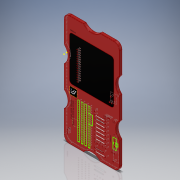
# Autodesk Inventor part: M5 Stack
Saved by Autodesk Inventor 2019 (Build 230136000, 136)
## iProperties
Created: 2020-01-20
Part Number: M5 Stack
Material: PET Plastic
Document SubType Name: Modeling
Designer: Leonardo
Density: 1.541 g/cm^3
Appearance: Red
Mass: 0.203324 g
Surface Area: 4.56566 cm^2
Volume: 0.199142 cm^3
Author: Leonardo
Autodesk Inventor part; units mm, degrees
(part 1 of 2)
ref_plane "YZ Plane" through (0, 0, 0) normal (1, 0, 0) x (0, 1, 0)
ref_plane "XZ Plane" through (0, 0, 0) normal (0, 1, 0) x (-1, 0, 0)
ref_plane "XY Plane" through (0, 0, 0) normal (0, 0, 1) x (1, 0, 0)
sketch "Sketch1" plane through (0, 0, 0) normal (0, 0, 1) x (1, 0, 0)
  line L0 (1, 6.5) -> (9, 6.5)
  line L1 (10, 5.5) -> (10, -12.5)
  line L2 (9, -13.5) -> (1, -13.5)
  line L3 (0, -12.5) -> (0, 5.5)
  arc A0 (10, 5.5) -> (9, 6.5) centre (9, 5.5) ccw
  arc A1 (1, 6.5) -> (0, 5.5) centre (1, 5.5) ccw
  arc A2 (0, -12.5) -> (1, -13.5) centre (1, -12.5) ccw
  arc A3 (9, -13.5) -> (10, -12.5) centre (9, -12.5) ccw
  point P0 (0, 0)
  point P1 (0, 6.5)
  point P2 (10, -13.5)
  point P3 (10, 6.5)
  point P4 (0, -13.5)
  dimension "d0" = 10
  dimension "d1" = 20
  dimension "d5" = 1
  dimension "d6" = 1
  dimension "d7" = 1
  constraints: 8 end point, 8 point on circle, 8 point on line, 8 tangent, 4 centre point, 2 parallel, 1 equal radius, 1 horizontal, 1 perpendicular
  measures "d0" distance of point (0, 6.5) point (10, 6.5)
  measures "d1" distance of point (10, 6.5) point (10, -13.5)
  measures "d5" radius of A0
  measures "d6" radius of A1
  measures "d7" radius of A2
extrude "Extrusion1" add sketch "Sketch1" along normal blind 0.5
sketch "Sketch3" plane through (0, 0, 0.5) normal (0, 0, 1) x (1, 0, 0)
  arc A0 (1, 6.5) -> (0, 5.5) centre (1, 5.5) ccw projected
  line L0 (1, 4) -> (9, 4)
  line L1 (9, 4) -> (9, -4.5)
  line L2 (9, -4.5) -> (1, -4.5)
  line L3 (1, -4.5) -> (1, 4)
  line L4 (9, -13.5) -> (1, -13.5) projected
  line L5 (5, -13.5) -> (5, -6)
  circle A1 centre (7.5, -6.0106) radius 0.0625
  line L6 (7.5, -6.0106) -> (7.5, -6.2106)
  line L7 (0, 5.5) -> (0, -12.5) projected
  line L8 (0, -3.5) -> (10.2754, -3.5)
  circle A2 centre (7.5, -6.2106) radius 0.0625
  line L9 (7.5, -6.2106) -> (7.5, -6.7106)
  circle A3 centre (7.5, -6.7106) radius 0.0625
  line L10 (7.5, -6.7106) -> (7.5, -7.2106)
  circle A4 centre (7.5, -7.2106) radius 0.0625
  circle A5 centre (7.5, -7.8356) radius 0.0625
  circle A6 centre (7.5, -8.4606) radius 0.0625
  circle A7 centre (7.5, -9.0856) radius 0.0625
  circle A8 centre (7.5, -9.7106) radius 0.0625
  circle A9 centre (7.5, -10.3356) radius 0.0625
  circle A10 centre (7.5, -10.9606) radius 0.0625
  line L11 (7.5, -5.9481) -> (5.5, -5.9481)
  line L12 (6.5, -5.9481) -> (6.5, -13.5)
  circle A11 centre (5.5, -6.0106) radius 0.0625
  line L13 (5.5, -6.0106) -> (5.5, -6.2106)
  circle A12 centre (5.5, -6.2106) radius 0.0625
  line L14 (5.5, -6.2106) -> (5.5, -6.7106)
  circle A13 centre (5.5, -6.7106) radius 0.0625
  line L15 (5.5, -6.7106) -> (5.5, -7.2106)
  circle A14 centre (5.5, -7.2106) radius 0.0625
  circle A15 centre (5.5, -7.8356) radius 0.0625
  line L16 (5.5, -7.7106) -> (5.5, -8.4606)
  circle A16 centre (5.5, -8.4606) radius 0.0625
  line L17 (5.5, -8.3356) -> (5.5, -9.0856)
  circle A17 centre (5.5, -9.0856) radius 0.0625
  line L18 (5.5, -8.9606) -> (5.5, -9.7106)
  circle A18 centre (5.5, -9.7106) radius 0.0625
  line L19 (5.5, -9.5856) -> (5.5, -10.3356)
  circle A19 centre (5.5, -10.3356) radius 0.0625
  line L20 (5.5, -10.2106) -> (5.5, -10.9606)
  circle A20 centre (5.5, -10.9606) radius 0.0625
  line L21 (5.5, -5.9481) -> (7.5, -5.9481)
  circle A21 centre (7.5, -12.3356) radius 0.0625
  circle A22 centre (5.5, -12.3356) radius 0.0625
  line L22 (7.5, -11.7731) -> (7.1, -11.7731)
  line L23 (7.5, -11.7731) -> (7.9, -11.7731) construction
  circle A23 centre (7.1, -11.7731) radius 0.0625
  line L24 (5.5, -10.9606) -> (5.5, -12.3782)
  line L25 (7.5, -11.0231) -> (7.7613, -11.0231)
  circle A24 centre (5.5, -11.7731) radius 0.0625
  circle A25 centre (6.5, -10.9606) radius 0.0625
  circle A26 centre (7, -10.9606) radius 0.0625
  circle A27 centre (6, -10.9606) radius 0.0625
  point P0 (0, 0)
  dimension "d10" = 0.125
  dimension "d35" = 0.125
  dimension "d8" = 7.5
  dimension "d11" = 0.2
  dimension "d12" = 0.125
  dimension "d13" = 1
  dimension "d14" = 8.5
  dimension "d15" = 8
  dimension "d16" = 0.5
  dimension "d17" = 0.125
  dimension "d18" = 0.5
  dimension "d19" = 0.125
  dimension "d23" = 0.125
  dimension "d25" = 0.125
  dimension "d27" = 0.125
  dimension "d29" = 0.125
  dimension "d31" = 0.125
  dimension "d38" = 2
  dimension "d64" = 0.5
  dimension "d65" = 0.5
  dimension "d66" = 0.5
  dimension "d67" = 0.5
  dimension "d68" = 0.5
  dimension "d69" = 0.5
  dimension "d70" = 0.125
  dimension "d71" = 1.25
  dimension "d72" = 180
  dimension "d73" = 0.125
  dimension "d75" = 0.4
  dimension "d78" = 0.75
  dimension "d79" = 0.125
  dimension "d80" = 0.125
  dimension "d81" = 0.125
  dimension "d82" = 0.125
  constraints: 48 end point, 24 centre point, 16 symmetric about line, 12 coincident, 6 vertical, 5 horizontal, 3 midpoint, 3 vertical alignment, 2 parallel, 2 perpendicular, 2 point on line, 1 collinear, 16 other
  measures "d8" distance of L5.start L5.end
  measures "d11" distance of L6.start L6.end
  measures "d12" diameter of A2
  measures "d13" distance from line of L7 L0.start
  measures "d14" distance from line of L2 L0.end
  measures "d15" distance of L0.end L0.start
  measures "d16" distance of L9.start L9.end
  measures "d17" diameter of A3
  measures "d18" distance of L10.start L10.end
  measures "d19" diameter of A4
  measures "d23" diameter of A5
  measures "d25" diameter of A6
  measures "d27" diameter of A7
  measures "d29" diameter of A8
  measures "d31" diameter of A9
  measures "d38" distance of L11.start L11.end
  measures "d70" diameter of A21
  measures "d72" angle of L22 L23
  measures "d73" diameter of A23
  measures "d75" distance of L22.end L22.start
  measures "d78" distance from line of L22.start L25
  measures "d79" diameter of A24
  measures "d80" diameter of A25
  measures "d81" diameter of A26
  measures "d82" diameter of A27
sketch "Sketch4" plane through (0, 0, 0.5) normal (0, 0, 1) x (1, 0, 0)
  line L0 (0, 5.5) -> (0, -12.5) projected
  line L1 (0, -3.5) -> (14.3961, -3.5)
  circle A0 centre (7.5, -8.4606) radius 0.0625 projected
  circle A1 centre (7.5, -6.0106) radius 0.0625 projected
  line L2 (7.5, -6.0106) -> (10.4645, -6.0106)
  line L3 (7.5, -6.0106) -> (10.4645, -6.0106) construction
  circle A2 centre (7.725, -6.0106) radius 0.0625
  circle A3 centre (7.95, -6.0106) radius 0.0625
  circle A4 centre (8.095, -6.0106) radius 0.0625
  circle A5 centre (8.24, -6.0106) radius 0.0625
  circle A6 centre (8.865, -6.0106) radius 0.0625
  circle A7 centre (9.09, -6.0106) radius 0.0625
  line L4 (9.09, -6.0106) -> (9.09, -8.5018)
  line L5 (9.09, -6.0106) -> (11.5812, -6.0106) construction
  circle A8 centre (9.09, -8.5018) radius 0.125
  line L6 (9.09, -8.5018) -> (9.09, -10.8899)
  line L7 (9.09, -8.5018) -> (11.4781, -8.5018) construction
  circle A9 centre (9.09, -8.9993) radius 0.0625
  circle A10 centre (9.09, -9.4343) radius 0.0625
  circle A11 centre (9.09, -9.8693) radius 0.0625
  circle A12 centre (9.09, -10.3668) radius 0.125
  line L8 (9.09, -10.8899) -> (9.09, -11.0971)
  line L9 (10, -12.5) -> (10, 5.5) projected
  circle A13 centre (9.0887, -11.003) radius 0.1
  circle A14 centre (8.6887, -11.003) radius 0.1
  line L10 (7.5, -12.3316) -> (9.6048, -12.3316)
  line L11 (7.5, -12.3316) -> (9.6048, -12.3316) construction
  line L12 (8.89, -11.003) -> (9.29, -11.003)
  circle A15 centre (8.8887, -12.3316) radius 0.1
  point P0 (0, 0)
  dimension "d41" = 0.125
  dimension "d42" = 0.1
  dimension "d43" = 0.125
  dimension "d44" = 0.125
  dimension "d45" = 0.125
  dimension "d46" = 0.1
  dimension "d47" = 0.02
  dimension "d48" = 0.02
  dimension "d49" = 0.125
  dimension "d50" = 0.125
  dimension "d51" = 0.1
  dimension "d52" = 0.5
  dimension "d53" = 90
  dimension "d54" = 0.25
  dimension "d55" = 90
  dimension "d56" = 0.125
  dimension "d57" = 0.125
  dimension "d58" = 0.125
  dimension "d59" = 0.25
  dimension "d60" = 0.31
  dimension "d61" = 0.31
  dimension "d62" = 0.31
  dimension "d63" = 0.31
  dimension "d84" = 0.2
  dimension "d86" = 0.2
  dimension "d87" = 0.2
  dimension "d90" = 0.2
  constraints: 22 end point, 14 centre point, 10 point on line, 6 horizontal, 4 equal length, 1 coincident, 1 midpoint, 1 parallel
  measures "d41" diameter of A2
  measures "d43" diameter of A3
  measures "d44" diameter of A4
  measures "d45" diameter of A5
  measures "d49" diameter of A6
  measures "d50" diameter of A7
  measures "d53" angle of L4 L5
  measures "d54" diameter of A8
  measures "d55" angle of L6 L7
  measures "d56" diameter of A9
  measures "d57" diameter of A10
  measures "d58" diameter of A11
  measures "d59" diameter of A12
  measures "d84" diameter of A13
  measures "d86" diameter of A14
  measures "d90" diameter of A15
extrude "Extrusion3" cut sketch "Sketch3" against normal blind 2 contours A1 | A4 | A3 L10 L9 | L9 L10 A3 | A2 L9 L6 | L6 L9 A2 | A25 L12 | L12 A25 | A14 | A13 L15 L14 | L14 L15 A13 | A12 L14 L13 | L13 L14 A12 | A11 | A5 | A6 | A7 | A8 | A9 | A10 | A15 L16 | A22 | A20 L24 L20 | L20 L24 A20 | A19 L20 L19 | L19 L20 A19 | A18 L19 L18 | L18 L19 A18 | A17 L18 L17 | L17 L18 A17 | A16 L17 L16 | L16 L17 A16 | L16 A15 | A21 | A23 | A26 | A27
extrude "Extrusion4" cut sketch "Sketch4" against normal blind 2 contours A13 L12 L8 | L8 L12 A13 | A12 L6 | L6 A12 | A11 L6 | L6 A11 | A10 L6 | L6 A10 | A9 L6 | L6 A9 | A8 L6 L4 | L4 L6 A8 | A7 L2 | L2 L4 A7 | A6 L2 | L2 A6 | A5 L2 | L2 A5 | A4 L2 | L2 A4 | A3 L2 | L2 A3 | A2 L2 | L2 A2 | L2 A7 L4 | L12 A13 | A14 | A15 L10 | L10 A15
sketch "Sketch5" plane through (0, 0, 0.5) normal (0, 0, 1) x (1, 0, 0)
  line L0 (0, -12.5) -> (10, -12.5)
  line L1 (0, -12.5) -> (10, -12.5) construction
  line L2 (5, -12.5) -> (5, -4)
  line L3 (5, -12.5) -> (2.2, -12.5)
  line L4 (2.2, -12.5) -> (2.2, -5.5)
  line L5 (2.2, -5.5) -> (2.2, -6)
  circle A0 centre (2.625, -6) radius 0.0625
  circle A1 centre (3.25, -6) radius 0.0625
  circle A2 centre (3.875, -6) radius 0.0625
  circle A3 centre (4.5, -6) radius 0.0625
  line L6 (2.625, -6) -> (2.625, -12.5)
  line L7 (2.625, -6) -> (9.125, -6) construction
  line L8 (2.625, -6.36) -> (2.9536, -6.36)
  line L9 (2.625, -6.72) -> (2.9536, -6.72)
  line L10 (2.625, -7.08) -> (3, -7.08)
  line L11 (2.625, -8.16) -> (3.0688, -8.16)
  line L12 (2.625, -8.52) -> (2.9536, -8.52)
  line L13 (2.625, -8.88) -> (3.3125, -8.88)
  line L14 (2.625, -9.24) -> (3.1875, -9.24)
  line L15 (2.625, -9.6) -> (3.25, -9.6)
  line L16 (2.625, -9.96) -> (3.3913, -9.96)
  line L17 (2.625, -10.32) -> (3.3125, -10.32)
  line L18 (2.625, -10.68) -> (3.1226, -10.68)
  line L19 (2.625, -11.04) -> (3.1226, -11.04)
  line L20 (2.625, -11.4) -> (3.1875, -11.4)
  line L21 (2.625, -11.76) -> (3.25, -11.76)
  line L22 (2.625, -12.12) -> (3.1875, -12.12)
  line L23 (2.625, -7.44) -> (3.0082, -7.44)
  line L24 (2.625, -7.8) -> (3.1226, -7.8)
  circle A4 centre (2.625, -6.36) radius 0.0625
  circle A5 centre (3.25, -6.36) radius 0.0625
  circle A6 centre (3.875, -6.36) radius 0.0625
  circle A7 centre (4.5, -6.36) radius 0.0625
  circle A8 centre (2.625, -6.72) radius 0.0625
  circle A9 centre (3.25, -6.72) radius 0.0625
  circle A10 centre (3.875, -6.72) radius 0.0625
  circle A11 centre (4.5, -6.72) radius 0.0625
  circle A12 centre (2.625, -7.08) radius 0.0625
  circle A13 centre (3.25, -7.08) radius 0.0625
  circle A14 centre (3.875, -7.08) radius 0.0625
  circle A15 centre (4.5, -7.08) radius 0.0625
  circle A16 centre (2.625, -7.44) radius 0.0625
  circle A17 centre (3.25, -7.44) radius 0.0625
  circle A18 centre (3.875, -7.44) radius 0.0625
  circle A19 centre (4.5, -7.44) radius 0.0625
  circle A20 centre (2.625, -7.8) radius 0.0625
  circle A21 centre (3.25, -7.8) radius 0.0625
  circle A22 centre (3.875, -7.8) radius 0.0625
  circle A23 centre (4.5, -7.8) radius 0.0625
  circle A24 centre (2.625, -8.16) radius 0.0625
  circle A25 centre (3.25, -8.16) radius 0.0625
  circle A26 centre (3.875, -8.16) radius 0.0625
  circle A27 centre (4.5, -8.16) radius 0.0625
  circle A28 centre (2.625, -8.52) radius 0.0625
  circle A29 centre (3.25, -8.52) radius 0.0625
  circle A30 centre (3.875, -8.52) radius 0.0625
  circle A31 centre (4.5, -8.52) radius 0.0625
  circle A32 centre (2.625, -8.88) radius 0.0625
  circle A33 centre (3.25, -8.88) radius 0.0625
  circle A34 centre (3.875, -8.88) radius 0.0625
  circle A35 centre (4.5, -8.88) radius 0.0625
  circle A36 centre (2.625, -9.24) radius 0.0625
  circle A37 centre (3.25, -9.24) radius 0.0625
  circle A38 centre (3.875, -9.24) radius 0.0625
  circle A39 centre (4.5, -9.24) radius 0.0625
  circle A40 centre (2.625, -9.6) radius 0.0625
  circle A41 centre (3.25, -9.6) radius 0.0625
  circle A42 centre (3.875, -9.6) radius 0.0625
  circle A43 centre (4.5, -9.6) radius 0.0625
  circle A44 centre (2.625, -9.96) radius 0.0625
  circle A45 centre (3.25, -9.96) radius 0.0625
  circle A46 centre (3.875, -9.96) radius 0.0625
  circle A47 centre (4.5, -9.96) radius 0.0625
  circle A48 centre (2.625, -10.32) radius 0.0625
  circle A49 centre (3.25, -10.32) radius 0.0625
  circle A50 centre (3.875, -10.32) radius 0.0625
  circle A51 centre (4.5, -10.32) radius 0.0625
  circle A52 centre (2.625, -10.68) radius 0.0625
  circle A53 centre (3.25, -10.68) radius 0.0625
  circle A54 centre (3.875, -10.68) radius 0.0625
  circle A55 centre (4.5, -10.68) radius 0.0625
  circle A56 centre (2.625, -11.04) radius 0.0625
  circle A57 centre (3.25, -11.04) radius 0.0625
  circle A58 centre (3.875, -11.04) radius 0.0625
  circle A59 centre (4.5, -11.04) radius 0.0625
  circle A60 centre (2.625, -11.4) radius 0.0625
  circle A61 centre (3.25, -11.4) radius 0.0625
  circle A62 centre (3.875, -11.4) radius 0.0625
  circle A63 centre (4.5, -11.4) radius 0.0625
  circle A64 centre (2.625, -11.76) radius 0.0625
  circle A65 centre (3.25, -11.76) radius 0.0625
  circle A66 centre (3.875, -11.76) radius 0.0625
  circle A67 centre (4.5, -11.76) radius 0.0625
  circle A68 centre (2.625, -12.12) radius 0.0625
  circle A69 centre (3.25, -12.12) radius 0.0625
  circle A70 centre (3.875, -12.12) radius 0.0625
  circle A71 centre (4.5, -12.12) radius 0.0625
  line L25 (2.625, -12.12) -> (0.625, -12.12)
  circle A72 centre (0.625, -12.12) radius 0.0625
  circle A73 centre (0.625, -11.895) radius 0.0625
  circle A74 centre (0.625, -11.67) radius 0.0625
  circle A75 centre (0.625, -11.445) radius 0.0625
  point P0 (0, 0)
  dimension "d96" = 2.8
  dimension "d97" = 7
  dimension "d99" = 0.5
  dimension "d100" = 0.125
  dimension "d101" = 0.125
  dimension "d102" = 0.125
  dimension "d103" = 0.125
  dimension "d109" = 0.5
  dimension "d110" = 0.5
  dimension "d111" = 0.5
  dimension "d112" = 0.5
  dimension "d114" = 6.5
  dimension "d115" = 0.36
  dimension "d116" = 0.36
  dimension "d117" = 0.36
  dimension "d118" = 0.36
  dimension "d119" = 0.36
  dimension "d120" = 0.36
  dimension "d121" = 0.36
  dimension "d122" = 0.36
  dimension "d124" = 0.36
  dimension "d125" = 0.36
  dimension "d126" = 0.36
  dimension "d127" = 0.36
  dimension "d128" = 0.36
  dimension "d129" = 0.36
  dimension "d130" = 0.36
  dimension "d131" = 0.36
  dimension "d132" = 0.36
  dimension "d133" = 0.125
  dimension "d134" = 0.125
  dimension "d135" = 0.125
  dimension "d136" = 0.125
  dimension "d137" = 0.5
  dimension "d138" = 0.5
  dimension "d139" = 0.5
  dimension "d140" = 0.125
  dimension "d141" = 0.125
  dimension "d142" = 0.125
  dimension "d143" = 0.125
  dimension "d144" = 0.5
  dimension "d145" = 0.5
  dimension "d146" = 0.5
  dimension "d147" = 0.125
  dimension "d148" = 0.125
  dimension "d149" = 0.125
  dimension "d150" = 0.125
  dimension "d151" = 0.5
  dimension "d152" = 0.5
  dimension "d153" = 0.5
  dimension "d154" = 0.125
  dimension "d155" = 0.125
  dimension "d156" = 0.125
  dimension "d157" = 0.125
  dimension "d158" = 0.5
  dimension "d159" = 0.5
  dimension "d160" = 0.5
  dimension "d161" = 0.125
  dimension "d162" = 0.125
  dimension "d163" = 0.125
  dimension "d164" = 0.125
  dimension "d165" = 0.5
  dimension "d166" = 0.5
  dimension "d167" = 0.5
  constraints: 76 centre point, 50 end point, 21 horizontal, 3 point on line, 1 coincident, 1 collinear, 1 midpoint, 1 perpendicular, 20 other
  measures "d96" distance of L2.start L3.end
  measures "d97" distance of L3.end L4.end
  measures "d99" distance of L4.end L5.end
  measures "d100" diameter of A0
  measures "d101" diameter of A1
  measures "d102" diameter of A2
  measures "d103" diameter of A3
  measures "d109" distance from line of L2 A3.centre
  measures "d114" distance of point (2.625, -12.5) L7.start
  measures "d115" distance of L8.start L7.start
  measures "d116" distance of L9.start L8.start
  measures "d117" distance of L9.start L10.start
  measures "d118" distance of L23.start L10.start
  measures "d119" distance of L24.start L23.start
  measures "d120" distance of L11.start L24.start
  measures "d121" distance of L12.start L11.start
  measures "d122" distance of L12.start L13.start
  measures "d124" distance of L14.start L13.start
  measures "d125" distance of L14.start L15.start
  measures "d126" distance of L15.start L16.start
  measures "d127" distance of L16.start L17.start
  measures "d128" distance of L17.start L18.start
  measures "d129" distance of L18.start L19.start
  measures "d130" distance of L20.start L19.start
  measures "d131" distance of L20.start L21.start
  measures "d132" distance of L21.start L22.start
  measures "d133" diameter of A4
  measures "d134" diameter of A5
  measures "d135" diameter of A6
  measures "d136" diameter of A7
  measures "d140" diameter of A8
  measures "d141" diameter of A9
  measures "d142" diameter of A10
  measures "d143" diameter of A11
  measures "d147" diameter of A12
  measures "d148" diameter of A13
  measures "d149" diameter of A14
  measures "d150" diameter of A15
  measures "d154" diameter of A16
  measures "d155" diameter of A17
  measures "d156" diameter of A18
  measures "d157" diameter of A19
  measures "d161" diameter of A20
  measures "d162" diameter of A21
  measures "d163" diameter of A22
  measures "d164" diameter of A23
extrude "Extrusion5" cut sketch "Sketch5" against normal blind 2 contours A72 | A0 | A4 L6 | L6 L8 A4 | A8 L6 | L6 L9 A8 | A12 L6 | L6 L10 A12 | A16 L6 | L6 L23 A16 | A20 L6 | L6 L24 A20 | A24 L6 | L6 L11 A24 | A28 L6 | L6 L12 A28 | A33 L13 | L13 A33 | A32 L6 | L6 L13 A32 | A37 | A36 L6 | L6 L14 A36 | A41 | A40 L6 | L6 L15 A40 | A45 L16 | L16 A45 | A44 L6 | L6 L16 A44 | A49 L17 | L17 A49 | A48 L6 | L6 L17 A48 | A52 L6 | L6 L18 A52 | A56 L6 | L6 L19 A56 | A61 | A60 L6 | L6 L20 A60 | A65 | A64 L6 | L6 L21 A64 | A69 | A68 L25 L6 | L6 L22 A68 | A68 L6 L25 | L6 A68 L22 | L6 A64 L21 | L6 A60 L20 | L6 A56 L19 | L6 A52 L18 | L6 A48 L17 | L6 A44 L16 | L6 A40 L15 | L6 A36 L14 | L6 A32 L13 | L6 A28 L12 | L6 A24 L11 | L6 A20 L24 | L6 A16 L23 | L6 A12 L10 | L6 A8 L9 | L6 A4 L8 | A1 | A2 | A3 | A5 | A6 | A7 | A9 | A10 | A11 | A13 | A14 | A15 | A17 | A18 | A19 | A21 | A22 | A23 | A25 | A26 | A27 | A29 | A30 | A31 | A34 | A35 | A38 | A39 | A42 | A43 | A46 | A47 | A50 | A51 | A53 | A54 | A55 | A57 | A58 | A59 | A62 | A63 | A66 | A67 | A70 | A71 | A73 | A74 | A75
sketch "Sketch6" plane through (0, 0, 0.5) normal (0, 0, 1) x (1, 0, 0)
  arc A0 (1, 6.5) -> (0, 5.5) centre (1, 5.5) ccw projected
  line L0 (1, 5.5) -> (1, 4)
  arc A1 (10, 5.5) -> (9, 6.5) centre (9, 5.5) ccw projected
  line L1 (9, 5.5) -> (9, 4)
  line L2 (1.5, 4) -> (8.5, 4)
  line L3 (1, 3.5) -> (1, -3.5)
  line L4 (9, 3.5) -> (9, -3.5)
  line L5 (8.5, -4) -> (1.5, -4)
  arc A2 (1.5, 4) -> (1, 3.5) centre (1.5, 3.5) ccw
  arc A3 (9, 3.5) -> (8.5, 4) centre (8.5, 3.5) ccw
  arc A4 (8.5, -4) -> (9, -3.5) centre (8.5, -3.5) ccw
  arc A5 (1, -3.5) -> (1.5, -4) centre (1.5, -3.5) ccw
  point P0 (0, 0)
  point P1 (1, -4)
  point P2 (9, -4)
  dimension "d262" = 1.5
  dimension "d263" = 1.5
  dimension "d264" = 8
  dimension "d265" = 8
  dimension "d266" = 0.5
  constraints: 12 end point, 8 point on circle, 8 point on line, 8 tangent, 4 centre point, 3 equal radius, 3 vertical, 1 perpendicular
  measures "d262" distance of L0.start L0.end
  measures "d263" distance of L1.start L1.end
  measures "d264" distance of L0.end point (1, -4)
  measures "d265" distance of L1.end point (9, -4)
  measures "d266" radius of A2
extrude "Extrusion6" add sketch "Sketch6" along normal blind 0.01
sketch "Sketch7" plane through (0, 0, 0.51) normal (0, 0, 1) x (1, 0, 0)
  arc A0 (1, -3.5) -> (1.5, -4) centre (1.5, -3.5) ccw projected
  line L0 (2.5, -3.5) -> (2.5, 4)
  line L1 (8.5, 4) -> (1.5, 4) projected
  line L2 (2.5, -3.14) -> (2.35, -3.14)
  line L3 (2.5, -3.1812) -> (2.65, -3.1812) construction
  line L4 (2.5, -2.78) -> (2.3618, -2.78)
  line L5 (2.5, -2.42) -> (2.4691, -2.42)
  line L6 (2.5, 4) -> (2.5, 2)
  line L7 (2.5, 2) -> (2, 2)
  line L8 (2.5, -2.06) -> (2.3278, -2.06)
  line L9 (2.5, -1.7) -> (2.3, -1.7)
  line L10 (2.5, -1.34) -> (2.2167, -1.34)
  line L11 (2.5, -0.98) -> (2.1573, -0.98)
  line L12 (2.5, -0.62) -> (2.276, -0.62)
  line L13 (2.5, -0.26) -> (2.3286, -0.26)
  line L14 (2.5, 0.1) -> (2.276, 0.1)
  line L15 (2.5, 0.46) -> (2.2167, 0.46)
  line L16 (2.5, 0.82) -> (2.276, 0.82)
  line L17 (2.5, 1.18) -> (2.3286, 1.18)
  line L18 (2.5, 1.54) -> (2.276, 1.54)
  line L19 (2.5, 1.9) -> (2.3, 1.9)
  circle A1 centre (2.5, -3.14) radius 0.05
  circle A2 centre (2.35, -3.14) radius 0.05
  circle A3 centre (2.5, -2.78) radius 0.05
  circle A4 centre (2.35, -2.78) radius 0.05
  circle A5 centre (2.5, -2.42) radius 0.05
  circle A6 centre (2.35, -2.42) radius 0.05
  circle A7 centre (2.5, -2.06) radius 0.05
  circle A8 centre (2.35, -2.06) radius 0.05
  circle A9 centre (2.5, -1.7) radius 0.05
  circle A10 centre (2.35, -1.7) radius 0.05
  circle A11 centre (2.5, -1.34) radius 0.05
  circle A12 centre (2.35, -1.34) radius 0.05
  circle A13 centre (2.5, -0.98) radius 0.05
  circle A14 centre (2.35, -0.98) radius 0.05
  circle A15 centre (2.5, -0.62) radius 0.05
  circle A16 centre (2.35, -0.62) radius 0.05
  circle A17 centre (2.5, -0.26) radius 0.05
  circle A18 centre (2.35, -0.26) radius 0.05
  circle A19 centre (2.5, 0.1) radius 0.05
  circle A20 centre (2.35, 0.1) radius 0.05
  circle A21 centre (2.5, 0.46) radius 0.05
  circle A22 centre (2.35, 0.46) radius 0.05
  circle A23 centre (2.5, 0.82) radius 0.05
  circle A24 centre (2.35, 0.82) radius 0.05
  circle A25 centre (2.5, 1.18) radius 0.05
  circle A26 centre (2.35, 1.18) radius 0.05
  circle A27 centre (2.5, 1.54) radius 0.05
  circle A28 centre (2.35, 1.54) radius 0.05
  circle A29 centre (2.5, 1.9) radius 0.05
  circle A30 centre (2.35, 1.9) radius 0.05
  point P0 (0, 0)
  dimension "d270" = 1.5
  dimension "d276" = 2
  dimension "d277" = 5.5
  dimension "d278" = 0.36
  dimension "d279" = 0.36
  dimension "d280" = 0.36
  dimension "d281" = 0.36
  dimension "d282" = 0.36
  dimension "d283" = 0.36
  dimension "d284" = 0.36
  dimension "d285" = 0.36
  dimension "d286" = 0.36
  dimension "d287" = 0.36
  dimension "d288" = 0.36
  dimension "d289" = 0.36
  dimension "d290" = 0.36
  dimension "d291" = 0.36
  dimension "d292" = 0.36
  dimension "d293" = 0.1
  dimension "d294" = 0.1
  dimension "d296" = 0.1
  dimension "d297" = 0.1
  dimension "d299" = 0.1
  dimension "d300" = 0.1
  dimension "d302" = 0.1
  dimension "d303" = 0.1
  dimension "d305" = 0.1
  dimension "d306" = 0.1
  dimension "d308" = 0.1
  dimension "d309" = 0.1
  dimension "d311" = 0.1
  dimension "d312" = 0.1
  dimension "d314" = 0.1
  dimension "d315" = 0.1
  dimension "d317" = 0.1
  dimension "d318" = 0.1
  dimension "d320" = 0.1
  dimension "d321" = 0.1
  dimension "d323" = 0.1
  dimension "d324" = 0.1
  dimension "d326" = 0.1
  dimension "d327" = 0.1
  dimension "d329" = 0.1
  dimension "d330" = 0.1
  dimension "d332" = 0.1
  dimension "d333" = 0.1
  dimension "d335" = 0.1
  dimension "d336" = 0.1
  constraints: 36 end point, 30 centre point, 16 horizontal, 1 point on line, 20 other
  measures "d270" distance of A0.start point (2.5, -3.5)
  measures "d276" distance of L6.start L6.end
  measures "d277" distance of point (2.5, -3.5) L6.end
  measures "d278" distance of L2.start point (2.5, -3.5)
  measures "d279" distance of L4.start L2.start
  measures "d280" distance of L5.start L4.start
  measures "d281" distance of L5.start L8.start
  measures "d282" distance of L8.start L9.start
  measures "d283" distance of L9.start L10.start
  measures "d284" distance of L10.start L11.start
  measures "d285" distance of L11.start L12.start
  measures "d286" distance of L12.start L13.start
  measures "d287" distance of L13.start L14.start
  measures "d288" distance of L14.start L15.start
  measures "d289" distance of L15.start L16.start
  measures "d290" distance of L16.start L17.start
  measures "d291" distance of L17.start L18.start
  measures "d292" distance of L18.start L19.start
  measures "d293" diameter of A1
  measures "d294" diameter of A2
  measures "d296" diameter of A3
  measures "d297" diameter of A4
  measures "d299" diameter of A5
  measures "d300" diameter of A6
  measures "d302" diameter of A7
  measures "d303" diameter of A8
  measures "d305" diameter of A9
  measures "d306" diameter of A10
  measures "d308" diameter of A11
  measures "d309" diameter of A12
  measures "d311" diameter of A13
  measures "d312" diameter of A14
  measures "d314" diameter of A15
  measures "d315" diameter of A16
  measures "d317" diameter of A17
  measures "d318" diameter of A18
  measures "d320" diameter of A19
  measures "d321" diameter of A20
  measures "d323" diameter of A21
  measures "d324" diameter of A22
  measures "d326" diameter of A23
  measures "d327" diameter of A24
  measures "d329" diameter of A25
  measures "d330" diameter of A26
  measures "d332" diameter of A27
  measures "d333" diameter of A28
  measures "d335" diameter of A29
  measures "d336" diameter of A30
extrude "Extrusion7" cut sketch "Sketch7" against normal blind 5
sketch "Sketch8" plane through (0, 0, 0.51) normal (0, 0, 1) x (1, 0, 0)
  circle A0 centre (2.5, -3.14) radius 0.05 projected
  line L0 (2.5, -3.14) -> (9, -3.1286)
  line L1 (2.5, -3.14) -> (9, -3.14) construction
  line L2 (8.4116, -3.14) -> (8.4104, -2.44)
  line L3 (8.4116, -3.14) -> (9.1116, -3.14) construction
  line L4 (8.4116, -3.14) -> (8.2116, -3.14)
  line L5 (8.2116, -3.14) -> (8.2121, -3.39)
  circle A1 centre (8.4104, -2.44) radius 0.1
  circle A2 centre (8.2121, -3.39) radius 0.1
  circle A3 centre (8.6121, -3.3893) radius 0.1
  point P0 (0, 0)
  dimension "d341" = 0.7
  dimension "d342" = 90.1
  dimension "d344" = 0.25
  dimension "d345" = 0.2
  dimension "d346" = 0.2
  dimension "d347" = 0.2
  constraints: 12 end point, 3 centre point, 2 coincident, 2 equal length, 2 horizontal, 2 perpendicular, 2 point on line, 1 symmetric about line, 1 other
  measures "d341" distance of L2.start L2.end
  measures "d342" angle of L3 L2
  measures "d344" distance of L4.end L5.end
  measures "d345" diameter of A1
  measures "d346" diameter of A2
extrude "Extrusion8" cut sketch "Sketch8" against normal blind 5 contours A1 | A2 | A3
sketch "Sketch9" plane through (0, 0, 0.5) normal (0, 0, 1) x (1, 0, 0)
  line L0 (9, 6.5) -> (1, 6.5) projected
  line L1 (1, 6.5) -> (9, 6.5)
  line L2 (5, 6.5) -> (6.5, 6.5)
  line L3 (5, 6.5) -> (3.5, 6.5)
  arc A0 (3.5, 6.5) -> (6.5, 6.5) centre (5, 7.8229) ccw
  line L4 (10, -12.5) -> (10, 5.5) projected
  line L5 (10, 5.5) -> (10, -12.5)
  line L6 (10, -7) -> (10, -5.5)
  line L7 (10, -7) -> (10, -8.5)
  arc A1 (10, -5.5) -> (10, -8.5) centre (11.3229, -7) ccw
  line L8 (10, 0) -> (10, 1.5)
  line L9 (10, 0) -> (10, -1.5)
  arc A2 (10, 1.5) -> (10, -1.5) centre (11.3229, 0) ccw
  line L10 (8.5, 4) -> (1.5, 4) projected
  line L11 (5, 4) -> (5, 2.9081)
  line L12 (9, -13.5) -> (1, -13.5) projected
  line L13 (5, -13.5) -> (6.5, -13.5)
  line L14 (5, -13.5) -> (3.5, -13.5)
  arc A3 (6.5, -13.5) -> (3.5, -13.5) centre (5, -14.8229) ccw
  arc A4 (0, -8.5) -> (0, -5.5) centre (-1.3229, -7) ccw
  arc A5 (0, -1.5) -> (0, 1.5) centre (-1.3229, 0) ccw
  line L15 (0, 1.5) -> (0, -1.5)
  line L16 (0, 5.5) -> (0, -12.5) projected
  line L17 (0, -5.5) -> (0, -8.5)
  line L18 (10, 1.5) -> (10, -1.5)
  line L19 (10, -5.5) -> (10, -8.5)
  line L20 (3.5, -13.5) -> (6.5, -13.5)
  line L21 (3.5, 6.5) -> (6.5, 6.5)
  point P0 (0, 0)
  dimension "d350" = 1.5
  dimension "d351" = 1.5
  dimension "d352" = 2
  dimension "d353" = 1.5
  dimension "d354" = 1.5
  dimension "d355" = 2
  dimension "d356" = 1.5
  dimension "d357" = 1.5
  dimension "d358" = 2
  dimension "d359" = 1.5
  dimension "d360" = 1.5
  dimension "d361" = 2
  constraints: 34 end point, 13 point on circle, 10 point on line, 6 centre point, 6 collinear, 6 symmetric about line, 3 midpoint, 2 vertical, 2 other
  measures "d350" distance of L2.start L3.end
  measures "d351" distance of L2.end L2.start
  measures "d352" radius of A0
  measures "d353" distance of L6.start L6.end
  measures "d354" distance of L6.start L7.end
  measures "d355" radius of A1
  measures "d356" distance of L8.start L8.end
  measures "d357" distance of L8.start L9.end
  measures "d358" radius of A2
  measures "d359" distance of L13.start L13.end
  measures "d360" distance of L13.start L14.end
  measures "d361" radius of A3
extrude "Extrusion9" cut sketch "Sketch9" against normal blind 5
sketch "Sketch10" plane through (0, 0, 0.5) normal (0, 0, 1) x (1, 0, 0)
  circle A0 centre (7.5, -6.0106) radius 0.0625 projected
  line L0 (7.5, -6.0106) -> (7.25, -6.0106)
  circle A1 centre (7.25, -6.0106) radius 0.0625
  line L1 (7.25, -6.0106) -> (7.25, -6.4106)
  circle A2 centre (7.25, -6.2106) radius 0.0625
  circle A3 centre (7.25, -6.4106) radius 0.0625
  arc A4 (10, 1.5) -> (10, -1.5) centre (11.3229, 0) ccw projected
  line L2 (10, -1.5) -> (9.5, -1.5)
  line L3 (9.5, -1.5) -> (9.5, -1.75)
  circle A5 centre (9.5, -1.75) radius 0.06
  line L4 (9.5, -1.75) -> (9.5, -2.0978)
  circle A6 centre (9.5, -1.945) radius 0.06
  point P0 (0, 0)
  dimension "d364" = 0.25
  dimension "d365" = 0.125
  dimension "d366" = 0.125
  dimension "d367" = 0.125
  dimension "d368" = 0.075
  dimension "d369" = 0.075
  dimension "d370" = 0.5
  dimension "d371" = 0.25
  dimension "d372" = 0.12
  dimension "d373" = 0.12
  dimension "d374" = 0.075
  constraints: 10 end point, 5 centre point, 3 coincident, 2 horizontal, 2 vertical, 1 midpoint, 1 perpendicular, 1 point on line
  measures "d364" distance of L0.start L0.end
  measures "d365" diameter of A1
  measures "d366" diameter of A2
  measures "d367" diameter of A3
  measures "d370" distance of L2.start L2.end
  measures "d371" distance of L2.end L3.end
  measures "d372" diameter of A5
  measures "d373" diameter of A6
extrude "Extrusion10" cut sketch "Sketch10" against normal blind 5 contours A3 | A2 L1 | L1 A2 | A1 L1 L0 | L0 L1 A1 | A5 L4 L3 | A6 L4 | L4 A6 | L3 L4 A5
sketch "Sketch11" plane through (0, 0, 0.5) normal (0, 0, 1) x (1, 0, 0)
  line L0 (2.3544, -4.4131) -> (2.3544, -5.7164) construction
  line L1 (2.3544, -5.7164) -> (1.0511, -5.7164) construction
  line L2 (1.0511, -5.7164) -> (1.0511, -4.4131) construction
  line L3 (1.0511, -4.4131) -> (2.3544, -4.4131) construction
  point P0 (0, 0)
  constraints: 2 other
sketch "Sketch12" plane through (0, 0, 0.5) normal (0, 0, 1) x (1, 0, 0)
  line L0 (1.7538, -6.4382) -> (1.7538, -12.3726) construction
  line L1 (1.7538, -12.3726) -> (1.0975, -12.3726) construction
  line L2 (1.0975, -12.3726) -> (1.0975, -6.4382) construction
  line L3 (1.0975, -6.4382) -> (1.7538, -6.4382) construction
  point P0 (0, 0)
  constraints: 2 other
sketch "Sketch13" plane through (0, 0, 0.5) normal (0, 0, 1) x (1, 0, 0)
  line L0 (0.8039, -10.9951) -> (1.2924, -10.9951) construction
  line L1 (1.2924, -10.9951) -> (1.2924, -11.2025) construction
  line L2 (1.2924, -11.2025) -> (0.8039, -11.2025) construction
  line L3 (0.8039, -11.2025) -> (0.8039, -10.9951) construction
  line L4 (1.109, 4.4654) -> (1.9804, 4.4654) construction
  line L5 (1.9804, 4.4654) -> (1.9804, 3.6467) construction
  line L6 (1.9804, 3.6467) -> (1.109, 3.6467) construction
  line L7 (1.109, 3.6467) -> (1.109, 4.4654) construction
  line L8 (8.7639, -6.173) -> (9.7984, -6.173) construction
  line L9 (9.7984, -6.173) -> (9.7984, -6.3814) construction
  line L10 (9.7984, -6.3814) -> (8.7639, -6.3814) construction
  line L11 (8.7639, -6.3814) -> (8.7639, -6.173) construction
  point P0 (0, 0)
  constraints: 6 other
sketch "Sketch14" plane through (0, 0, 0.5) normal (0, 0, 1) x (1, 0, 0)
  line L0 (7.4146, -5.8096) -> (7.5723, -5.8096) construction
  line L1 (7.5723, -5.8096) -> (7.5723, -5.9135) construction
  line L2 (7.5723, -5.9135) -> (7.4146, -5.9135) construction
  line L3 (7.4146, -5.9135) -> (7.4146, -5.8096) construction
  line L4 (7.3691, -6.3733) -> (7.5675, -6.3733) construction
  line L5 (7.5675, -6.3733) -> (7.5675, -6.4805) construction
  line L6 (7.5675, -6.4805) -> (7.3691, -6.4805) construction
  line L7 (7.3691, -6.4805) -> (7.3691, -6.3733) construction
  line L8 (7.883, -6.359) -> (8.4288, -6.359) construction
  line L9 (8.4288, -6.359) -> (8.4288, -6.6227) construction
  line L10 (8.4288, -6.6227) -> (7.883, -6.6227) construction
  line L11 (7.883, -6.6227) -> (7.883, -6.359) construction
  line L12 (8.4882, -8.419) -> (8.4882, -9.5555) construction
  line L13 (8.4882, -9.5555) -> (8.2751, -9.5555) construction
  line L14 (8.2751, -9.5555) -> (8.2751, -8.419) construction
  line L15 (8.2751, -8.419) -> (8.4882, -8.419) construction
  line L16 (8.9627, -8.0088) -> (9.2158, -8.0088) construction
  line L17 (9.2158, -8.0088) -> (9.2158, -8.1396) construction
  line L18 (9.2158, -8.1396) -> (8.9627, -8.1396) construction
  line L19 (8.9627, -8.1396) -> (8.9627, -8.0088) construction
  line L20 (2.5597, -5.6716) -> (2.692, -5.6716) construction
  line L21 (2.692, -5.6716) -> (2.692, -5.773) construction
  line L22 (2.692, -5.773) -> (2.5597, -5.773) construction
  line L23 (2.5597, -5.773) -> (2.5597, -5.6716) construction
  line L24 (3.1701, -5.6641) -> (3.3024, -5.6641) construction
  line L25 (3.3024, -5.6641) -> (3.3024, -5.7655) construction
  line L26 (3.3024, -5.7655) -> (3.1701, -5.7655) construction
  line L27 (3.1701, -5.7655) -> (3.1701, -5.6641) construction
  line L28 (3.7951, -5.758) -> (3.7951, -5.6567) construction
  line L29 (3.7951, -5.6567) -> (3.9274, -5.6567) construction
  line L30 (3.9274, -5.6567) -> (3.9274, -5.758) construction
  line L31 (3.9274, -5.758) -> (3.7951, -5.758) construction
  line L32 (4.4349, -5.7579) -> (4.4349, -5.6565) construction
  line L33 (4.4349, -5.6565) -> (4.5672, -5.6565) construction
  line L34 (4.5672, -5.6565) -> (4.5672, -5.7579) construction
  line L35 (4.5672, -5.7579) -> (4.4349, -5.7579) construction
  point P0 (0, 0)
  constraints: 18 other
fillet "Fillet1" radius 0.05 40 edges at (7.75, 6.5, 0.5) (10, 3.5, 0.5) (9.7071, 6.2071, 0.5) (9.7071, 6.2071, 0) (7.75, 6.5, 0) (10, 3.5, 0) (9.3229, 0, 0.5) (9.3229, 0, 0) (10, -3.5, 0.5) (10, -3.5, 0) (9.3229, -7, 0.5) (9.3229, -7, 0) (9.7071, -13.2071, 0.5) (7.75, -13.5, 0.5) (10, -10.5, 0.5) (9.7071, -13.2071, 0) (7.75, -13.5, 0) (10, -10.5, 0) (5, -12.8229, 0.5) (5, -12.8229, 0) (0.2929, -13.2071, 0.5) (0, -10.5, 0.5) (2.25, -13.5, 0.5) (0.2929, -13.2071, 0) (0, -10.5, 0) (2.25, -13.5, 0) (0.6771, -7, 0.5) (0.6771, -7, 0) (0, -3.5, 0) (0, -3.5, 0.5) (0.6771, 0, 0.5) (0.6771, 0, 0) (0.2929, 6.2071, 0.5) (2.25, 6.5, 0.5) (0, 3.5, 0.5) (0.2929, 6.2071, 0) (2.25, 6.5, 0) (0, 3.5, 0) (5, 5.8229, 0.5) (5, 5.8229, 0)
sketch "Sketch15" plane through (0, 0, 0.5) normal (0, 0, 1) x (1, 0, 0)
  line L0 (2.02, -5.9608) -> (2.297, -5.9608) construction
  line L1 (2.297, -5.9608) -> (2.297, -6.0645) construction
  line L2 (2.297, -6.0645) -> (2.02, -6.0645) construction
  line L3 (2.02, -6.0645) -> (2.02, -5.9608) construction
  line L4 (2.0248, -6.324) -> (2.2997, -6.324) construction
  line L5 (2.2997, -6.324) -> (2.2997, -6.4282) construction
  line L6 (2.2997, -6.4282) -> (2.0248, -6.4282) construction
  line L7 (2.0248, -6.4282) -> (2.0248, -6.324) construction
  line L8 (2.027, -6.6668) -> (2.272, -6.6668) construction
  line L9 (2.272, -6.6668) -> (2.272, -6.8384) construction
  line L10 (2.272, -6.8384) -> (2.027, -6.8384) construction
  line L11 (2.027, -6.8384) -> (2.027, -6.6668) construction
  point P0 (0, 0)
  constraints: 6 other
sketch "Sketch16" plane through (0, 0, 0.5) normal (0, 0, 1) x (1, 0, 0)
  line L0 (4.7602, -7.0192) -> (4.9953, -7.0192) construction
  line L1 (4.9953, -7.0192) -> (4.9953, -7.1195) construction
  line L2 (4.9953, -7.1195) -> (4.7602, -7.1195) construction
  line L3 (4.7602, -7.1195) -> (4.7602, -7.0192) construction
  line L4 (4.7564, -7.3862) -> (4.9915, -7.3862) construction
  line L5 (4.9915, -7.3862) -> (4.9915, -7.4865) construction
  line L6 (4.9915, -7.4865) -> (4.7564, -7.4865) construction
  line L7 (4.7564, -7.4865) -> (4.7564, -7.3862) construction
  line L8 (4.7526, -7.7334) -> (4.9877, -7.7334) construction
  line L9 (4.9877, -7.7334) -> (4.9877, -7.8337) construction
  line L10 (4.9877, -7.8337) -> (4.7526, -7.8337) construction
  line L11 (4.7526, -7.8337) -> (4.7526, -7.7334) construction
  line L12 (4.7468, -8.4756) -> (4.982, -8.4756) construction
  line L13 (4.982, -8.4756) -> (4.982, -8.576) construction
  line L14 (4.982, -8.576) -> (4.7468, -8.576) construction
  line L15 (4.7468, -8.576) -> (4.7468, -8.4756) construction
  line L16 (4.7626, -8.0841) -> (4.9978, -8.0841) construction
  line L17 (4.9978, -8.0841) -> (4.9978, -8.1992) construction
  line L18 (4.9978, -8.1992) -> (4.7626, -8.1992) construction
  line L19 (4.7626, -8.1992) -> (4.7626, -8.0841) construction
  line L20 (4.7635, -6.8509) -> (4.9986, -6.8509) construction
  line L21 (4.9986, -6.8509) -> (4.9986, -6.9512) construction
  line L22 (4.9986, -6.9512) -> (4.7635, -6.9512) construction
  line L23 (4.7635, -6.9512) -> (4.7635, -6.8509) construction
  point P0 (0, 0)
  constraints: 12 other
sketch "Sketch17" plane through (0, 0, 0) normal (0, 0, -1) x (-1, 0, 0)
  line L0 (-0.9859, -9.6669) -> (-0.9859, -10.7764) construction
  line L1 (-0.9859, -10.7764) -> (-2.0954, -10.7764) construction
  line L2 (-2.0954, -10.7764) -> (-2.0954, -9.6669) construction
  line L3 (-2.0954, -9.6669) -> (-0.9859, -9.6669) construction
  line L4 (-1.552, -9.5021) -> (-1.552, -6) construction
  line L5 (-1.552, -6) -> (-1, -6) construction
  line L6 (-1, -6) -> (-1, -9.5021) construction
  line L7 (-1, -9.5021) -> (-1.552, -9.5021) construction
  point P0 (0, 0)
  constraints: 4 other
sketch "Sketch18" plane through (0, 0, 0) normal (0, 0, -1) x (-1, 0, 0)
  line L0 (-9.5923, -1.442) -> (-8.9408, -1.442) construction
  line L1 (-8.9408, -1.442) -> (-8.9408, -1.5748) construction
  line L2 (-8.9408, -1.5748) -> (-9.5923, -1.5748) construction
  line L3 (-9.5923, -1.5748) -> (-9.5923, -1.442) construction
  line L4 (-7.3221, -5.8086) -> (-6.8476, -5.8086) construction
  line L5 (-6.8476, -5.8086) -> (-6.8476, -5.9124) construction
  line L6 (-6.8476, -5.9124) -> (-7.3221, -5.9124) construction
  line L7 (-7.3221, -5.9124) -> (-7.3221, -5.8086) construction
  point P0 (0, 0)
  constraints: 4 other